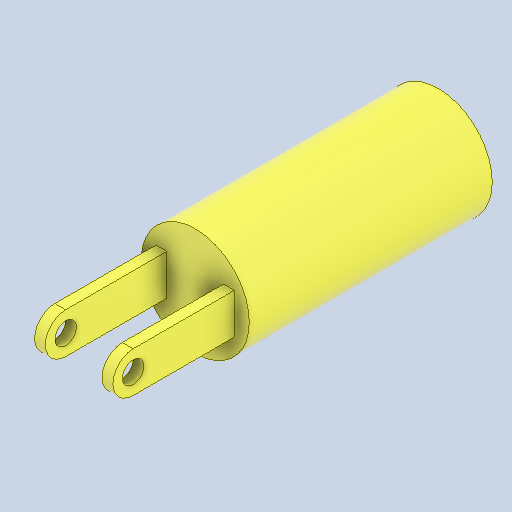
# Autodesk Inventor part: 节块
Saved by Autodesk Inventor 2022 (Build 260153000, 153)
## iProperties
Created: 2023-02-24
Part Number: 节块
Material: 常规
Document SubType Name: Modeling
Designer: 李承轩
Density: 1 g/cm^3
Appearance: 平滑 - 黄色
Author: 李承轩
Autodesk Inventor part; units mm, degrees
ref_plane "YZ Plane" through (0, 0, 0) normal (1, 0, 0) x (0, 1, 0)
ref_plane "XZ Plane" through (0, 0, 0) normal (0, 1, 0) x (-1, 0, 0)
ref_plane "XY Plane" through (0, 0, 0) normal (0, 0, 1) x (1, 0, 0)
sketch "草图1" plane through (0, 0, 0) normal (0, 0, 1) x (1, 0, 0)
  circle A0 centre (0, 0) radius 20 projected
  circle A1 centre (0, 0) radius 10 projected
  point P0 (0, 0)
extrude "拉伸1" add sketch "草图1" along normal blind 40 contours A0 | A1
sketch "草图2" plane through (0, 0, 40) normal (0, 0, 1) x (1, 0, 0)
  circle A0 centre (0, 0) radius 20 projected
  point P0 (0, 0)
extrude "拉伸2" add sketch "草图2" along normal blind 50
sketch "草图3" plane through (0, 0, 90) normal (0, 0, 1) x (1, 0, 0)
  line L0 (0, 0) -> (0, 22.0262)
  line L1 (-10.5, -7.5) -> (-14.5, -7.5)
  line L2 (-14.5, -7.5) -> (-14.5, 7.5)
  line L3 (-14.5, 7.5) -> (-10.5, 7.5)
  line L4 (-10.5, 7.5) -> (-10.5, -7.5)
  line L5 (-10.5, -7.5) -> (-14.5, 7.5) construction
  line L6 (-14.5, -7.5) -> (-10.5, 7.5) construction
  line L7 (10.5, -7.5) -> (14.5, -7.5)
  line L8 (14.5, -7.5) -> (14.5, 7.5)
  line L9 (14.5, 7.5) -> (10.5, 7.5)
  line L10 (10.5, 7.5) -> (10.5, -7.5)
  line L11 (10.5, -7.5) -> (14.5, 7.5) construction
  line L12 (14.5, -7.5) -> (10.5, 7.5) construction
  point P0 (-12.5, 0)
  point P1 (12.5, 0)
  point P2 (-12.5, 0)
  dimension "d4" = 25
  dimension "d5" = 4
  dimension "d6" = 15
  constraints: 26 end point, 5 midpoint, 5 symmetric about line, 2 parallel, 1 horizontal, 1 horizontal alignment, 1 perpendicular, 1 vertical
  measures "d4" distance of point (12.5, 0) point (-12.5, 0)
  measures "d5" distance of L2.end L3.end
  measures "d6" distance of L3.end L1.start
extrude "拉伸3" add sketch "草图3" along normal blind 45
full round fillet "全圆角1" first side at (-13.1667, -7.5, 105) centre faces at (-11.8333, -2.5, 135) second side at (-11.8333, 7.5, 105)
full round fillet "全圆角2" first side at (13.1667, 7.5, 105) centre faces at (13.1667, -2.5, 135) second side at (11.8333, -7.5, 105)
sketch "草图4" plane through (-14.5, -7.5, 90) normal (-1, 0, 0) x (0, 0, 1)
  arc A0 (37.5, 0) -> (37.5, 15) centre (37.5, 7.5) ccw projected
  point P0 (-90, 7.5)
  constraints: 1 coincident
hole "孔1" at (-14.5, 0, 127.5) direction (1, 0, 0) diameter 8 end through all
sketch "草图5" plane through (0, 0, 0) normal (0, 0, -1) x (-1, 0, 0)
  circle A0 centre (0, 0) radius 20 projected
  point P0 (0, 0)
  constraints: 1 coincident
hole "孔2" at (0, 0, 0) direction (0, 0, 1) diameter 20 depth 40
